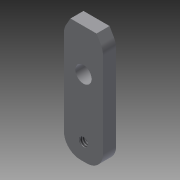
# Autodesk Inventor part: plate_02 for metal
Saved by Autodesk Inventor 2015 (Build 190159000, 159)
## iProperties
Created: 2013-12-02
Part Number: plate_02 for metal
Material: Generic
Document SubType Name: Modeling
Designer: Labadmin
Density: 1 g/cm^3
Appearance: Default
Author: Labadmin
Autodesk Inventor part; units mm, degrees
ref_plane "YZ Plane" through (0, 0, 0) normal (1, 0, 0) x (0, 1, 0)
ref_plane "XZ Plane" through (0, 0, 0) normal (0, 1, 0) x (-1, 0, 0)
ref_plane "XY Plane" through (0, 0, 0) normal (0, 0, 1) x (1, 0, 0)
sketch "Sketch1" plane through (0, 0, 0) normal (0, 0, 1) x (1, 0, 0)
  line L0 (-5.334, 0) -> (5.334, 0) projected
  line L1 (0, -4.572) -> (0, 27.432) projected
  line L2 (3.81, 0) -> (-3.81, 0)
  line L3 (-3.81, 0) -> (-3.81, 20.6603)
  line L4 (3.81, 20.6603) -> (3.81, 0)
  line L5 (-3.81, 20.6603) -> (-2.54, 22.86)
  line L6 (-2.54, 22.86) -> (2.54, 22.86)
  line L7 (2.54, 22.86) -> (3.81, 20.6603)
  point P0 (0, 0)
  point P1 (0, 0)
  point P2 (0, 22.86)
  dimension "d0" = 22.86
  dimension "d1" = 5.08
  dimension "d2" = 60
  dimension "d3" = 7.62
  constraints: 12 end point, 3 midpoint, 2 perpendicular, 2 point on line, 1 horizontal, 1 horizontal alignment, 1 parallel
  measures "d0" distance between parallel lines of L0 L6
  measures "d1" distance of L5.end L6.end
  measures "d2" angle of L5 L6
  measures "d3" distance between parallel lines of L4 L3
extrude "Extrusion1" add sketch "Sketch1" against normal blind 2.54
sketch "Sketch2" plane through (0, 0, 0) normal (0, 0, 1) x (1, 0, 0)
  line L0 (0, -4.572) -> (0, 27.432) projected
  line L1 (2.54, 22.86) -> (-2.54, 22.86) projected
  point P0 (0, 0)
  point P1 (0, 14.7066)
  dimension "d18" = 8.1534
  constraints: 1 point on line
  measures "d18" vertical distance of L1.start point (0, 14.707)
hole "Hole1" at (0, 14.7066, 0) direction (0, 0, -1) diameter 3.175 end through all
fillet "Fillet1" radius 3.175 4 edges at (3.81, 0, -1.27) (-3.81, 0, -1.27) (3.81, 20.6603, -1.27) (-3.81, 20.6603, -1.27)
sketch "Sketch3" plane through (0, 0, 0) normal (0, 0, 1) x (1, 0, 0)
  point P0 (0, 0)
  point P1 (0, 3.302)
  dimension "d31" = 3.302
  measures "d31" distance of point (0, 0) point (0, 3.302)
hole "Hole3" at (0, 3.302, 0) direction (0, 0, -1) diameter 1.7018 end through all
body "Solid1"
